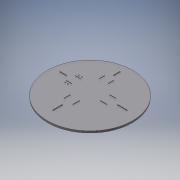
# Autodesk Inventor part: BallBallerina_BasePlate_v1
Saved by Autodesk Inventor 2016 (Build 200138000, 138)
## iProperties
Created: 2016-04-07
Part Number: BallBallerina_BasePlate_v1
Material: Generic
Document SubType Name: Modeling
Designer: Admin
Density: 1 g/cm^3
Appearance: Default
Author: Admin
Autodesk Inventor part; units mm, degrees
ref_plane "YZ Plane" through (0, 0, 0) normal (1, 0, 0) x (0, 1, 0)
ref_plane "XZ Plane" through (0, 0, 0) normal (0, 1, 0) x (-1, 0, 0)
ref_plane "XY Plane" through (0, 0, 0) normal (0, 0, 1) x (1, 0, 0)
sketch "Sketch1" plane through (0, 0, 0) normal (0, 0, 1) x (1, 0, 0)
  line L0 (-204.47, 0) -> (204.47, 0) projected
  line L1 (0, -204.47) -> (0, 204.47) projected
  circle A0 centre (0, 0) radius 146.05
  dimension "d0" = 292.1
  constraints: 1 centre point, 1 coincident
  measures "d0" diameter of A0
extrude "Extrusion1" add sketch "Sketch1" along normal blind 6
sketch "Sketch2" plane through (0, 0, 6) normal (0, 0, 1) x (1, 0, 0)
  circle A0 centre (0, 0) radius 114.3 construction
  arc A1 (-1.4999, 88.8873) -> (1.4999, 88.8873) centre (0, 0) ccw construction
  line L0 (-204.47, 0) -> (204.47, 0) construction
  line L1 (0, -204.47) -> (0, 204.47) construction
  arc A2 (1.4999, 114.2873) -> (-1.5, 114.2902) centre (0, 114.3) ccw
  arc A3 (-1.5, 88.9098) -> (1.4999, 88.9127) centre (0, 88.9) ccw
  line L2 (1.4999, 114.2902) -> (1.4999, 88.8873)
  line L3 (-1.5, 88.8873) -> (-1.5, 114.2902)
  arc A4 (-114.2873, 1.4999) -> (-114.2902, -1.5) centre (-114.3, 0) ccw
  arc A5 (-88.9098, -1.5) -> (-88.9127, 1.4999) centre (-88.9, 0) ccw
  line L4 (-114.2902, 1.4999) -> (-88.8873, 1.4999)
  line L5 (-88.8873, -1.5) -> (-114.2902, -1.5)
  arc A6 (-1.4999, -114.2873) -> (1.5, -114.2902) centre (0, -114.3) ccw
  arc A7 (1.5, -88.9098) -> (-1.4999, -88.9127) centre (0, -88.9) ccw
  line L6 (-1.4999, -114.2902) -> (-1.4999, -88.8873)
  line L7 (1.5, -88.8873) -> (1.5, -114.2902)
  arc A8 (88.9098, 1.5) -> (88.9127, -1.4999) centre (88.9, 0) ccw
  line L8 (88.8873, 1.5) -> (114.2902, 1.5)
  arc A9 (114.2873, -1.4999) -> (114.2902, 1.5) centre (114.3, 0) ccw
  line L9 (114.2902, -1.4999) -> (88.8873, -1.4999)
  point P0 (-88.8873, -1.4999)
  point P1 (1.4999, -88.8873)
  point P2 (88.8873, 1.4999)
  dimension "d3" = 228.6
  dimension "d4" = 177.8
  dimension "d5" = 3
  dimension "d6" = 3
  dimension "d13" = 3
  dimension "d14" = 3
  dimension "d15" = 3
  dimension "d16" = 3
  dimension "d17" = 3
  dimension "d18" = 3
  constraints: 24 point on circle, 16 end point, 14 point on line, 10 centre point, 4 parallel, 2 coincident
  measures "d3" diameter of A0
  measures "d4" diameter of A1
  measures "d5" diameter of A2
  measures "d6" diameter of A3
  measures "d13" diameter of A4
  measures "d14" diameter of A5
  measures "d15" diameter of A6
  measures "d16" diameter of A7
  measures "d17" diameter of A9
  measures "d18" diameter of A8
extrude "Extrusion2" cut sketch "Sketch2" against normal blind 6
sketch "Sketch4" plane through (0, 0, 6) normal (0, 0, 1) x (1, 0, 0)
  line L0 (-204.47, 0) -> (204.47, 0) projected
  line L1 (0, -204.47) -> (0, 204.47) projected
  line L2 (-17, 70) -> (-15, 70)
  line L3 (-15, 70) -> (-15, 50)
  line L4 (-15, 50) -> (-17, 50)
  line L5 (-17, 50) -> (-17, 70)
  line L6 (17, 70) -> (15, 70)
  line L7 (15, 70) -> (15, 50)
  line L8 (15, 50) -> (17, 50)
  line L9 (17, 50) -> (17, 70)
  line L10 (-17, -70) -> (-15, -70)
  line L11 (-15, -70) -> (-15, -50)
  line L12 (-15, -50) -> (-17, -50)
  line L13 (-17, -50) -> (-17, -70)
  line L14 (17, -70) -> (15, -70)
  line L15 (15, -70) -> (15, -50)
  line L16 (15, -50) -> (17, -50)
  line L17 (17, -50) -> (17, -70)
  line L18 (-70, -17) -> (-70, -15)
  line L19 (-70, -15) -> (-50, -15)
  line L20 (-50, -15) -> (-50, -17)
  line L21 (-50, -17) -> (-70, -17)
  line L22 (-70, 17) -> (-70, 15)
  line L23 (-70, 15) -> (-50, 15)
  line L24 (-50, 15) -> (-50, 17)
  line L25 (-50, 17) -> (-70, 17)
  line L26 (70, -17) -> (70, -15)
  line L27 (70, -15) -> (50, -15)
  line L28 (50, -15) -> (50, -17)
  line L29 (50, -17) -> (70, -17)
  line L30 (70, 17) -> (70, 15)
  line L31 (70, 15) -> (50, 15)
  line L32 (50, 15) -> (50, 17)
  line L33 (50, 17) -> (70, 17)
  point P0 (0, 0)
  dimension "d21" = 2
  dimension "d22" = 50
  dimension "d23" = 20
  dimension "d24" = 15
  dimension "d25" = 2
  dimension "d26" = 20
  constraints: 64 end point, 12 symmetric about line, 4 parallel, 2 perpendicular, 1 horizontal
  measures "d21" distance of L3.end L4.end
  measures "d22" distance between parallel lines of L0 L4
  measures "d23" distance between parallel lines of L2 L4
  measures "d24" distance between parallel lines of L1 L3
  measures "d25" distance of L20.start L20.end
  measures "d26" distance between parallel lines of L18 L20
extrude "Extrusion3" cut sketch "Sketch4" against normal blind 6
sketch "Sketch5" plane through (0, 0, 0) normal (0, 0, -1) x (-1, 0, 0)
  circle A0 centre (66, 24.11) radius 1.75
  circle A1 centre (54, 24.11) radius 1.75
  circle A2 centre (54.9574, -24.11) radius 1.75
  circle A3 centre (64.9809, -24.11) radius 1.75
  point P0 (0, 0)
  constraints: 4 centre point, 8 other
extrude "Extrusion4" cut sketch "Sketch5" against normal blind 10
body "Solid1"
